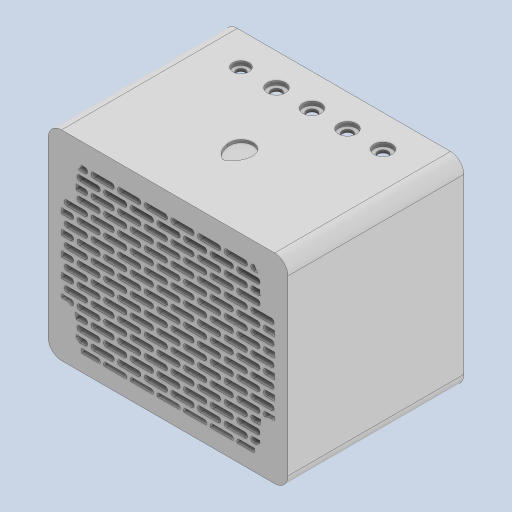
# Autodesk Inventor part: caixa_central
Saved by Autodesk Inventor 2023 (Build 270158000, 158)
## iProperties
Created: 2023-03-03
Part Number: caixa_central
Material: Genérico
Document SubType Name: Modeling
Designer: texugo
Density: 1 g/cm^3
Appearance: Padrão
Author: texugo
Autodesk Inventor part; units mm, degrees
(part 1 of 7)
ref_plane "YZ Plane" through (0, 0, 0) normal (1, 0, 0) x (0, 1, 0)
ref_plane "XZ Plane" through (0, 0, 0) normal (0, 1, 0) x (-1, 0, 0)
ref_plane "XY Plane" through (0, 0, 0) normal (0, 0, 1) x (1, 0, 0)
sketch "Esboço1" plane through (0, 0, 0) normal (0, 0, 1) x (1, 0, 0)
  line L0 (-75, 70) -> (75, 70)
  line L1 (85, 60) -> (85, -60)
  line L2 (75, -70) -> (-75, -70)
  line L3 (-85, -60) -> (-85, 60)
  line L4 (85, 70) -> (-85, -70) construction
  line L5 (-78, 73) -> (78, 73)
  line L6 (88, 63) -> (88, -63)
  line L7 (78, -73) -> (-78, -73)
  line L8 (-88, -63) -> (-88, 63)
  line L9 (-88, 73) -> (88, -73) construction
  arc A0 (-75, 70) -> (-85, 60) centre (-75, 60) ccw
  arc A1 (-78, 73) -> (-88, 63) centre (-78, 63) ccw
  arc A2 (85, 60) -> (75, 70) centre (75, 60) ccw
  arc A3 (88, 63) -> (78, 73) centre (78, 63) ccw
  arc A4 (75, -70) -> (85, -60) centre (75, -60) ccw
  arc A5 (78, -73) -> (88, -63) centre (78, -63) ccw
  arc A6 (-88, -63) -> (-78, -73) centre (-78, -63) ccw
  arc A7 (-85, -60) -> (-75, -70) centre (-75, -60) ccw
  circle A8 centre (-73.7339, -61.8573) radius 1.25
  line L10 (0, 0) -> (0, 1.4904)
  line L11 (0, 0) -> (1.3651, 0)
  line L12 (-73.7339, -52.8401) -> (-85, -52.8401)
  line L13 (-64.7396, -62.5) -> (-64.7396, -70)
  arc A9 (-64.7396, -62.5) -> (-74.5, -52.8727) centre (-73.7339, -61.8573) ccw
  circle A10 centre (73.7339, -61.8573) radius 1.25
  line L14 (73.7339, -52.8401) -> (85, -52.8401)
  line L15 (64.7396, -62.5) -> (64.7396, -70)
  arc A11 (74.5, -52.8727) -> (64.7396, -62.5) centre (73.7339, -61.8573) ccw
  line L16 (-80, -42) -> (-77, -42)
  circle A12 centre (-77, -42) radius 1.25
  arc A13 (-69.0044, -42.2652) -> (-77, -34) centre (-77, -42) ccw
  line L17 (-77, -34) -> (-85, -34)
  line L18 (-69, -42) -> (-69, -54.1827)
  circle A14 centre (77, -42) radius 1.25
  arc A15 (77, -34) -> (69.0044, -42.2652) centre (77, -42) ccw
  line L19 (69, -42) -> (69, -54.1827)
  arc A16 (-77, 34) -> (-69.0044, 42.2652) centre (-77, 42) ccw
  line L20 (-77, 34) -> (-85, 34)
  line L21 (-69, 42) -> (-69, 54.1827)
  arc A17 (69.0044, 42.2652) -> (77, 34) centre (77, 42) ccw
  line L22 (69, 42) -> (69, 54.1827)
  line L23 (77, -34) -> (85, -34)
  circle A18 centre (-73.7339, 61.8573) radius 1.25
  line L24 (-73.7339, 52.8401) -> (-85, 52.8401)
  line L25 (-64.7396, 62.5) -> (-64.7396, 70)
  arc A19 (-74.5, 52.8727) -> (-64.7396, 62.5) centre (-73.7339, 61.8573) ccw
  arc A20 (64.7396, 62.5) -> (74.5, 52.8727) centre (73.7339, 61.8573) ccw
  line L26 (64.7396, 62.5) -> (64.7396, 70)
  line L27 (73.7339, 52.8401) -> (85, 52.8401)
  circle A21 centre (73.7339, 61.8573) radius 1.25
  line L28 (77, 34) -> (85, 34)
  circle A22 centre (-73.7339, 61.8573) radius 1.25
  circle A23 centre (73.7339, 61.8573) radius 1.25
  circle A24 centre (-77, 42) radius 1.25
  circle A25 centre (77, 42) radius 1.25
  dimension "d4" = 10
  dimension "d8" = 2.5
  dimension "d12" = 3
  dimension "d13" = 2.5
  constraints: 58 end point, 44 symmetric about line, 41 point on circle, 26 centre point, 20 tangent, 11 point on line, 7 coincident, 7 equal radius, 5 perpendicular, 4 parallel, 3 horizontal, 2 midpoint, 2 vertical, 14 other
  measures "d4" radius of A0
  measures "d8" diameter of A8
  measures "d12" distance of L16.start L16.end
  measures "d13" diameter of A12
extrude "Extrusão1" add sketch "Esboço1" along normal blind 4 contours L0 L25 A19 L24 L3 A0 | L0 L26 A20 L22 A17 L28 L1 L23 A15 L19 A11 L15 L2 L13 A9 L18 A13 L17 L3 L20 A16 L21 A19 L25 | L0 A2 L1 L27 A20 L26 | L24 A19 L21 A16 L20 L3 | A20 L27 L1 L28 A17 L22 | L17 A13 L18 A9 L12 L3 | L12 A9 L13 L2 A7 L3 | L1 L14 A11 L19 A15 L23 | L1 A4 L2 L15 A11 L14 | L5 A3 L6 A5 L7 A6 L8 A1 | A8 | A10 | A12 | A14 | A18 | A21 | A24 | A25
sketch "Esboço2" plane through (0, 0, 0) normal (0, 0, -1) x (-1, 0, 0)
  line L0 (-75, 70) -> (75, 70)
  line L1 (85, 60) -> (85, -60)
  line L2 (75, -70) -> (-75, -70)
  line L3 (-85, -60) -> (-85, 60)
  line L4 (85, 70) -> (-85, -70) construction
  line L5 (-78, 73) -> (78, 73)
  line L6 (88, 63) -> (88, -63)
  line L7 (78, -73) -> (-78, -73)
  line L8 (-88, -63) -> (-88, 63)
  line L9 (-88, 73) -> (88, -73) construction
  arc A0 (-75, 70) -> (-85, 60) centre (-75, 60) ccw
  arc A1 (-78, 73) -> (-88, 63) centre (-78, 63) ccw
  arc A2 (85, 60) -> (75, 70) centre (75, 60) ccw
  arc A3 (88, 63) -> (78, 73) centre (78, 63) ccw
  arc A4 (75, -70) -> (85, -60) centre (75, -60) ccw
  arc A5 (78, -73) -> (88, -63) centre (78, -63) ccw
  arc A6 (-88, -63) -> (-78, -73) centre (-78, -63) ccw
  arc A7 (-85, -60) -> (-75, -70) centre (-75, -60) ccw
  circle A8 centre (-73.7339, -61.8573) radius 1.25
  line L10 (0, 0) -> (0, 1.4904)
  line L11 (0, 0) -> (1.3651, 0)
  line L12 (-73.7339, -52.8401) -> (-85, -52.8401)
  line L13 (-64.7396, -62.5) -> (-64.7396, -70)
  arc A9 (-64.7396, -62.5) -> (-74.5, -52.8727) centre (-73.7339, -61.8573) ccw
  arc A10 (74.5, -52.8727) -> (64.7396, -62.5) centre (73.7339, -61.8573) ccw
  line L14 (64.7396, -62.5) -> (64.7396, -70)
  line L15 (73.7339, -52.8401) -> (85, -52.8401)
  circle A11 centre (73.7339, -61.8573) radius 1.25
  line L16 (-80, -42) -> (-77, -42)
  circle A12 centre (-77, -42) radius 1.25
  arc A13 (-69.0044, -42.2652) -> (-77, -34) centre (-77, -42) ccw
  line L17 (-77, -34) -> (-85, -34)
  line L18 (-69, -42) -> (-69, -54.1827)
  arc A14 (77, -34) -> (69.0044, -42.2652) centre (77, -42) ccw
  line L19 (69, -42) -> (69, -54.1827)
  circle A15 centre (77, -42) radius 1.25
  line L20 (-77, 34) -> (-85, 34)
  arc A16 (-77, 34) -> (-69.0044, 42.2652) centre (-77, 42) ccw
  line L21 (-69, 42) -> (-69, 54.1827)
  line L22 (69, 42) -> (69, 54.1827)
  arc A17 (69.0044, 42.2652) -> (77, 34) centre (77, 42) ccw
  line L23 (77, -34) -> (85, -34)
  line L24 (77, 34) -> (85, 34)
  line L25 (64.7396, 62.5) -> (64.7396, 70)
  arc A18 (64.7396, 62.5) -> (74.5, 52.8727) centre (73.7339, 61.8573) ccw
  line L26 (73.7339, 52.8401) -> (85, 52.8401)
  circle A19 centre (73.7339, 61.8573) radius 1.25
  line L27 (-64.7396, 62.5) -> (-64.7396, 70)
  arc A20 (-74.5, 52.8727) -> (-64.7396, 62.5) centre (-73.7339, 61.8573) ccw
  circle A21 centre (-73.7339, 61.8573) radius 1.25
  line L28 (-73.7339, 52.8401) -> (-85, 52.8401)
  circle A22 centre (-73.7339, 61.8573) radius 1.25
  circle A23 centre (73.7339, 61.8573) radius 1.25
  circle A24 centre (77, 42) radius 1.25
  circle A25 centre (-77, 42) radius 1.25
  dimension "d16" = 10
  dimension "d17" = 2.5
  dimension "d18" = 3
  dimension "d19" = 2.5
  constraints: 58 end point, 44 symmetric about line, 41 point on circle, 26 centre point, 20 tangent, 11 point on line, 7 coincident, 7 equal radius, 5 perpendicular, 4 parallel, 3 horizontal, 2 midpoint, 2 vertical, 14 other
  measures "d16" radius of A0
  measures "d17" diameter of A8
  measures "d18" distance of L16.start L16.end
  measures "d19" diameter of A12
extrude "Extrusão2" add sketch "Esboço2" along normal blind 10 contours L0 L27 A20 L28 L3 A0 | L0 A2 L1 L26 A18 L25 | L28 A20 L21 A16 L20 L3 | A18 L26 L1 L24 A17 L22 | L17 A13 L18 A9 L12 L3 | L12 A9 L13 L2 A7 L3 | L1 L15 A10 L19 A14 L23 | L1 A4 L2 L14 A10 L15 | L5 A3 L6 A5 L7 A6 L8 A1 | A8 | A11 | A12 | A15 | A19 | A21 | A24 | A25
sketch "Esboço3" plane through (0, 0, -10) normal (0, 0, -1) x (-1, 0, 0)
  line L0 (-75, 70) -> (75, 70)
  line L1 (85, 60) -> (85, -60)
  line L2 (75, -70) -> (-75, -70)
  line L3 (-85, -60) -> (-85, 60)
  line L4 (85, 70) -> (-85, -70) construction
  line L5 (-78, 73) -> (78, 73)
  line L6 (88, 63) -> (88, -63)
  line L7 (78, -73) -> (-78, -73)
  line L8 (-88, -63) -> (-88, 63)
  line L9 (-88, 73) -> (88, -73) construction
  arc A0 (-75, 70) -> (-85, 60) centre (-75, 60) ccw
  arc A1 (-78, 73) -> (-88, 63) centre (-78, 63) ccw
  arc A2 (85, 60) -> (75, 70) centre (75, 60) ccw
  arc A3 (88, 63) -> (78, 73) centre (78, 63) ccw
  arc A4 (75, -70) -> (85, -60) centre (75, -60) ccw
  arc A5 (78, -73) -> (88, -63) centre (78, -63) ccw
  arc A6 (-88, -63) -> (-78, -73) centre (-78, -63) ccw
  arc A7 (-85, -60) -> (-75, -70) centre (-75, -60) ccw
  circle A8 centre (-73.7339, -61.8573) radius 1.25
  line L10 (0, 0) -> (0, 1.4904)
  line L11 (0, 0) -> (1.3651, 0)
  line L12 (-73.7339, -52.8401) -> (-85, -52.8401)
  line L13 (-64.7396, -62.5) -> (-64.7396, -70)
  arc A9 (-64.7396, -62.5) -> (-74.5, -52.8727) centre (-73.7339, -61.8573) ccw
  arc A10 (74.5, -52.8727) -> (64.7396, -62.5) centre (73.7339, -61.8573) ccw
  line L14 (64.7396, -62.5) -> (64.7396, -70)
  line L15 (73.7339, -52.8401) -> (85, -52.8401)
  circle A11 centre (73.7339, -61.8573) radius 1.25
  line L16 (-80, -42) -> (-77, -42)
  circle A12 centre (-77, -42) radius 1.25
  arc A13 (-69.0044, -42.2652) -> (-77, -34) centre (-77, -42) ccw
  line L17 (-77, -34) -> (-85, -34)
  line L18 (-69, -42) -> (-69, -54.1827)
  arc A14 (77, -34) -> (69.0044, -42.2652) centre (77, -42) ccw
  line L19 (69, -42) -> (69, -54.1827)
  circle A15 centre (77, -42) radius 1.25
  line L20 (-77, 34) -> (-85, 34)
  arc A16 (-77, 34) -> (-69.0044, 42.2652) centre (-77, 42) ccw
  line L21 (-69, 42) -> (-69, 54.1827)
  line L22 (69, 42) -> (69, 54.1827)
  arc A17 (69.0044, 42.2652) -> (77, 34) centre (77, 42) ccw
  line L23 (77, -34) -> (85, -34)
  line L24 (77, 34) -> (85, 34)
  line L25 (64.7396, 62.5) -> (64.7396, 70)
  arc A18 (64.7396, 62.5) -> (74.5, 52.8727) centre (73.7339, 61.8573) ccw
  line L26 (73.7339, 52.8401) -> (85, 52.8401)
  circle A19 centre (73.7339, 61.8573) radius 1.25
  line L27 (-64.7396, 62.5) -> (-64.7396, 70)
  arc A20 (-74.5, 52.8727) -> (-64.7396, 62.5) centre (-73.7339, 61.8573) ccw
  circle A21 centre (-73.7339, 61.8573) radius 1.25
  line L28 (-73.7339, 52.8401) -> (-85, 52.8401)
  circle A22 centre (-73.7339, 61.8573) radius 1.25
  circle A23 centre (73.7339, 61.8573) radius 1.25
  circle A24 centre (77, 42) radius 1.25
  circle A25 centre (-77, 42) radius 1.25
  dimension "d22" = 10
  dimension "d23" = 2.5
  dimension "d24" = 3
  dimension "d25" = 2.5
  constraints: 58 end point, 44 symmetric about line, 41 point on circle, 26 centre point, 20 tangent, 11 point on line, 7 coincident, 7 equal radius, 5 perpendicular, 4 parallel, 3 horizontal, 2 midpoint, 2 vertical, 14 other
  measures "d22" radius of A0
  measures "d23" diameter of A8
  measures "d24" distance of L16.start L16.end
  measures "d25" diameter of A12
extrude "Extrusão3" cut sketch "Esboço3" against normal blind 5 contours A12 | A15 | A24 | A25
sketch "Esboço4" plane through (0, 0, -10) normal (0, 0, -1) x (-1, 0, 0)
  line L0 (-75, 70) -> (75, 70)
  line L1 (85, 60) -> (85, -60)
  line L2 (75, -70) -> (-75, -70)
  line L3 (-85, -60) -> (-85, 60)
  line L4 (85, 70) -> (-85, -70) construction
  line L5 (-78, 73) -> (78, 73)
  line L6 (88, 63) -> (88, -63)
  line L7 (78, -73) -> (-78, -73)
  line L8 (-88, -63) -> (-88, 63)
  line L9 (-88, 73) -> (88, -73) construction
  arc A0 (-75, 70) -> (-85, 60) centre (-75, 60) ccw
  arc A1 (-78, 73) -> (-88, 63) centre (-78, 63) ccw
  arc A2 (85, 60) -> (75, 70) centre (75, 60) ccw
  arc A3 (88, 63) -> (78, 73) centre (78, 63) ccw
  arc A4 (75, -70) -> (85, -60) centre (75, -60) ccw
  arc A5 (78, -73) -> (88, -63) centre (78, -63) ccw
  arc A6 (-88, -63) -> (-78, -73) centre (-78, -63) ccw
  arc A7 (-85, -60) -> (-75, -70) centre (-75, -60) ccw
  circle A8 centre (-73.7339, -61.8573) radius 1.25
  line L10 (0, 0) -> (0, 1.4904)
  line L11 (0, 0) -> (1.3651, 0)
  line L12 (-73.7339, -52.8401) -> (-85, -52.8401)
  line L13 (-64.7396, -62.5) -> (-64.7396, -70)
  arc A9 (-64.7396, -62.5) -> (-74.5, -52.8727) centre (-73.7339, -61.8573) ccw
  arc A10 (74.5, -52.8727) -> (64.7396, -62.5) centre (73.7339, -61.8573) ccw
  line L14 (64.7396, -62.5) -> (64.7396, -70)
  line L15 (73.7339, -52.8401) -> (85, -52.8401)
  circle A11 centre (73.7339, -61.8573) radius 1.25
  line L16 (-80, -42) -> (-77, -42)
  circle A12 centre (-77, -42) radius 1.25
  arc A13 (-69.0044, -42.2652) -> (-77, -34) centre (-77, -42) ccw
  line L17 (-77, -34) -> (-85, -34)
  line L18 (-69, -42) -> (-69, -54.1827)
  arc A14 (77, -34) -> (69.0044, -42.2652) centre (77, -42) ccw
  line L19 (69, -42) -> (69, -54.1827)
  circle A15 centre (77, -42) radius 1.25
  line L20 (-77, 34) -> (-85, 34)
  arc A16 (-77, 34) -> (-69.0044, 42.2652) centre (-77, 42) ccw
  line L21 (-69, 42) -> (-69, 54.1827)
  line L22 (69, 42) -> (69, 54.1827)
  arc A17 (69.0044, 42.2652) -> (77, 34) centre (77, 42) ccw
  line L23 (77, -34) -> (85, -34)
  line L24 (77, 34) -> (85, 34)
  line L25 (64.7396, 62.5) -> (64.7396, 70)
  arc A18 (64.7396, 62.5) -> (74.5, 52.8727) centre (73.7339, 61.8573) ccw
  line L26 (73.7339, 52.8401) -> (85, 52.8401)
  circle A19 centre (73.7339, 61.8573) radius 1.25
  line L27 (-64.7396, 62.5) -> (-64.7396, 70)
  arc A20 (-74.5, 52.8727) -> (-64.7396, 62.5) centre (-73.7339, 61.8573) ccw
  circle A21 centre (-73.7339, 61.8573) radius 1.25
  line L28 (-73.7339, 52.8401) -> (-85, 52.8401)
  circle A22 centre (-73.7339, 61.8573) radius 1.25
  circle A23 centre (73.7339, 61.8573) radius 1.25
  circle A24 centre (77, 42) radius 1.25
  circle A25 centre (-77, 42) radius 1.25
  dimension "d28" = 10
  dimension "d29" = 2.5
  dimension "d30" = 3
  dimension "d31" = 2.5
  constraints: 58 end point, 44 symmetric about line, 41 point on circle, 26 centre point, 20 tangent, 11 point on line, 7 coincident, 7 equal radius, 5 perpendicular, 4 parallel, 3 horizontal, 2 midpoint, 2 vertical, 14 other
  measures "d28" radius of A0
  measures "d29" diameter of A8
  measures "d30" distance of L16.start L16.end
  measures "d31" diameter of A12
extrude "Extrusão4" add sketch "Esboço4" along normal blind 70 contours L0 L27 A20 L28 L3 A0 | L0 A2 L1 L26 A18 L25 | L12 A9 L13 L2 A7 L3 | L1 A4 L2 L14 A10 L15 | L5 A3 L6 A5 L7 A6 L8 A1 | A8 | A11 | A19 | A21
sketch "Esboço5" plane through (0, 0, -80) normal (0, 0, -1) x (-1, 0, 0)
  line L0 (-75, 70) -> (75, 70)
  line L1 (85, 60) -> (85, -60)
  line L2 (75, -70) -> (-75, -70)
  line L3 (-85, -60) -> (-85, 60)
  line L4 (85, 70) -> (-85, -70) construction
  line L5 (-78, 73) -> (78, 73)
  line L6 (88, 63) -> (88, -63)
  line L7 (78, -73) -> (-78, -73)
  line L8 (-88, -63) -> (-88, 63)
  line L9 (-88, 73) -> (88, -73) construction
  arc A0 (-75, 70) -> (-85, 60) centre (-75, 60) ccw
  arc A1 (-78, 73) -> (-88, 63) centre (-78, 63) ccw
  arc A2 (85, 60) -> (75, 70) centre (75, 60) ccw
  arc A3 (88, 63) -> (78, 73) centre (78, 63) ccw
  arc A4 (75, -70) -> (85, -60) centre (75, -60) ccw
  arc A5 (78, -73) -> (88, -63) centre (78, -63) ccw
  arc A6 (-88, -63) -> (-78, -73) centre (-78, -63) ccw
  arc A7 (-85, -60) -> (-75, -70) centre (-75, -60) ccw
  circle A8 centre (-73.7339, -61.8573) radius 1.25
  line L10 (0, 0) -> (0, 1.4904)
  line L11 (0, 0) -> (1.3651, 0)
  line L12 (-73.7339, -52.8401) -> (-85, -52.8401)
  line L13 (-64.7396, -62.5) -> (-64.7396, -70)
  arc A9 (-64.7396, -62.5) -> (-74.5, -52.8727) centre (-73.7339, -61.8573) ccw
  arc A10 (74.5, -52.8727) -> (64.7396, -62.5) centre (73.7339, -61.8573) ccw
  line L14 (64.7396, -62.5) -> (64.7396, -70)
  line L15 (73.7339, -52.8401) -> (85, -52.8401)
  circle A11 centre (73.7339, -61.8573) radius 1.25
  line L16 (-80, -42) -> (-77, -42)
  circle A12 centre (-77, -42) radius 1.25
  arc A13 (-69.0044, -42.2652) -> (-77, -34) centre (-77, -42) ccw
  line L17 (-77, -34) -> (-85, -34)
  line L18 (-69, -42) -> (-69, -54.1827)
  arc A14 (77, -34) -> (69.0044, -42.2652) centre (77, -42) ccw
  line L19 (69, -42) -> (69, -54.1827)
  circle A15 centre (77, -42) radius 1.25
  line L20 (-77, 34) -> (-85, 34)
  arc A16 (-77, 34) -> (-69.0044, 42.2652) centre (-77, 42) ccw
  line L21 (-69, 42) -> (-69, 54.1827)
  line L22 (69, 42) -> (69, 54.1827)
  arc A17 (69.0044, 42.2652) -> (77, 34) centre (77, 42) ccw
  line L23 (77, -34) -> (85, -34)
  line L24 (77, 34) -> (85, 34)
  line L25 (64.7396, 62.5) -> (64.7396, 70)
  arc A18 (64.7396, 62.5) -> (74.5, 52.8727) centre (73.7339, 61.8573) ccw
  line L26 (73.7339, 52.8401) -> (85, 52.8401)
  circle A19 centre (73.7339, 61.8573) radius 1.25
  line L27 (-64.7396, 62.5) -> (-64.7396, 70)
  arc A20 (-74.5, 52.8727) -> (-64.7396, 62.5) centre (-73.7339, 61.8573) ccw
  circle A21 centre (-73.7339, 61.8573) radius 1.25
  line L28 (-73.7339, 52.8401) -> (-85, 52.8401)
  circle A22 centre (-73.7339, 61.8573) radius 1.25
  circle A23 centre (73.7339, 61.8573) radius 1.25
  circle A24 centre (77, 42) radius 1.25
  circle A25 centre (-77, 42) radius 1.25
  dimension "d34" = 10
  dimension "d35" = 2.5
  dimension "d36" = 3
  dimension "d37" = 2.5
  constraints: 58 end point, 44 symmetric about line, 41 point on circle, 26 centre point, 20 tangent, 11 point on line, 7 coincident, 7 equal radius, 5 perpendicular, 4 parallel, 3 horizontal, 2 midpoint, 2 vertical, 14 other
  measures "d34" radius of A0
  measures "d35" diameter of A8
  measures "d36" distance of L16.start L16.end
  measures "d37" diameter of A12
extrude "Extrusão5" cut sketch "Esboço5" against normal blind 7 contours A8 | A11 | A19 | A21
sketch "Esboço6" plane through (0, 0, -80) normal (0, 0, -1) x (-1, 0, 0)
  line L0 (-75, 70) -> (75, 70)
  line L1 (85, 60) -> (85, -60)
  line L2 (75, -70) -> (-75, -70)
  line L3 (-85, -60) -> (-85, 60)
  line L4 (85, 70) -> (-85, -70) construction
  line L5 (-78, 73) -> (78, 73)
  line L6 (88, 63) -> (88, -63)
  line L7 (78, -73) -> (-78, -73)
  line L8 (-88, -63) -> (-88, 63)
  line L9 (-88, 73) -> (88, -73) construction
  arc A0 (-75, 70) -> (-85, 60) centre (-75, 60) ccw
  arc A1 (-78, 73) -> (-88, 63) centre (-78, 63) ccw
  arc A2 (85, 60) -> (75, 70) centre (75, 60) ccw
  arc A3 (88, 63) -> (78, 73) centre (78, 63) ccw
  arc A4 (75, -70) -> (85, -60) centre (75, -60) ccw
  arc A5 (78, -73) -> (88, -63) centre (78, -63) ccw
  arc A6 (-88, -63) -> (-78, -73) centre (-78, -63) ccw
  arc A7 (-85, -60) -> (-75, -70) centre (-75, -60) ccw
  circle A8 centre (-73.7339, -61.8573) radius 1.25
  line L10 (0, 0) -> (0, 1.4904)
  line L11 (0, 0) -> (1.3651, 0)
  line L12 (-73.7339, -52.8401) -> (-85, -52.8401)
  line L13 (-64.7396, -62.5) -> (-64.7396, -70)
  arc A9 (-64.7396, -62.5) -> (-74.5, -52.8727) centre (-73.7339, -61.8573) ccw
  arc A10 (74.5, -52.8727) -> (64.7396, -62.5) centre (73.7339, -61.8573) ccw
  line L14 (64.7396, -62.5) -> (64.7396, -70)
  line L15 (73.7339, -52.8401) -> (85, -52.8401)
  circle A11 centre (73.7339, -61.8573) radius 1.25
  line L16 (-80, -42) -> (-77, -42)
  circle A12 centre (-77, -42) radius 1.25
  arc A13 (-69.0044, -42.2652) -> (-77, -34) centre (-77, -42) ccw
  line L17 (-77, -34) -> (-85, -34)
  line L18 (-69, -42) -> (-69, -54.1827)
  arc A14 (77, -34) -> (69.0044, -42.2652) centre (77, -42) ccw
  line L19 (69, -42) -> (69, -54.1827)
  circle A15 centre (77, -42) radius 1.25
  line L20 (-77, 34) -> (-85, 34)
  arc A16 (-77, 34) -> (-69.0044, 42.2652) centre (-77, 42) ccw
  line L21 (-69, 42) -> (-69, 54.1827)
  line L22 (69, 42) -> (69, 54.1827)
  arc A17 (69.0044, 42.2652) -> (77, 34) centre (77, 42) ccw
  line L23 (77, -34) -> (85, -34)
  line L24 (77, 34) -> (85, 34)
  line L25 (64.7396, 62.5) -> (64.7396, 70)
  arc A18 (64.7396, 62.5) -> (74.5, 52.8727) centre (73.7339, 61.8573) ccw
  line L26 (73.7339, 52.8401) -> (85, 52.8401)
  circle A19 centre (73.7339, 61.8573) radius 1.25
  line L27 (-64.7396, 62.5) -> (-64.7396, 70)
  arc A20 (-74.5, 52.8727) -> (-64.7396, 62.5) centre (-73.7339, 61.8573) ccw
  circle A21 centre (-73.7339, 61.8573) radius 1.25
  line L28 (-73.7339, 52.8401) -> (-85, 52.8401)
  circle A22 centre (-73.7339, 61.8573) radius 1.25
  circle A23 centre (73.7339, 61.8573) radius 1.25
  circle A24 centre (77, 42) radius 1.25
  circle A25 centre (-77, 42) radius 1.25
  dimension "d40" = 10
  dimension "d41" = 2.5
  dimension "d42" = 3
  dimension "d43" = 2.5
  constraints: 58 end point, 44 symmetric about line, 41 point on circle, 26 centre point, 20 tangent, 11 point on line, 7 coincident, 7 equal radius, 5 perpendicular, 4 parallel, 3 horizontal, 2 midpoint, 2 vertical, 14 other
  measures "d40" radius of A0
  measures "d41" diameter of A8
  measures "d42" distance of L16.start L16.end
  measures "d43" diameter of A12
extrude "Extrusão6" add sketch "Esboço6" along normal blind 45 contours L5 A3 L6 A5 L7 A6 L8 A1
sketch "Esboço7" plane through (0, 0, 0) normal (0, 0, 1) x (1, 0, 0)
  line L0 (80, 75) -> (-80, 75)
  line L1 (-90, 65) -> (-90, -65)
  line L2 (-80, -75) -> (80, -75)
  line L3 (90, -65) -> (90, 65)
  line L4 (90, 75) -> (-90, -75) construction
  line L5 (-90, 75) -> (90, -75) construction
  arc A0 (80, -75) -> (90, -65) centre (80, -65) ccw
  arc A1 (-90, -65) -> (-80, -75) centre (-80, -65) ccw
  arc A2 (-80, 75) -> (-90, 65) centre (-80, 65) ccw
  arc A3 (90, 65) -> (80, 75) centre (80, 65) ccw
  line L6 (-75, 70) -> (75, 70)
  line L7 (85, 60) -> (85, -60)
  line L8 (75, -70) -> (-75, -70)
  line L9 (-85, -60) -> (-85, 60)
  line L10 (85, 70) -> (-85, -70) construction
  line L11 (-78, 73) -> (78, 73)
  line L12 (88, 63) -> (88, -63)
  line L13 (78, -73) -> (-78, -73)
  line L14 (-88, -63) -> (-88, 63)
  line L15 (-88, 73) -> (88, -73) construction
  arc A4 (-75, 70) -> (-85, 60) centre (-75, 60) ccw
  arc A5 (-78, 73) -> (-88, 63) centre (-78, 63) ccw
  arc A6 (85, 60) -> (75, 70) centre (75, 60) ccw
  arc A7 (88, 63) -> (78, 73) centre (78, 63) ccw
  arc A8 (75, -70) -> (85, -60) centre (75, -60) ccw
  arc A9 (78, -73) -> (88, -63) centre (78, -63) ccw
  arc A10 (-88, -63) -> (-78, -73) centre (-78, -63) ccw
  arc A11 (-85, -60) -> (-75, -70) centre (-75, -60) ccw
  circle A12 centre (-73.7339, -61.8573) radius 1.25
  line L16 (0, 0) -> (0, 1.4904)
  line L17 (0, 0) -> (1.3651, 0)
  line L18 (-73.7339, -52.8401) -> (-85, -52.8401)
  line L19 (-64.7396, -62.5) -> (-64.7396, -70)
  arc A13 (-64.7396, -62.5) -> (-74.5, -52.8727) centre (-73.7339, -61.8573) ccw
  arc A14 (74.5, -52.8727) -> (64.7396, -62.5) centre (73.7339, -61.8573) ccw
  line L20 (64.7396, -62.5) -> (64.7396, -70)
  line L21 (73.7339, -52.8401) -> (85, -52.8401)
  circle A15 centre (73.7339, -61.8573) radius 1.25
  line L22 (-80, -42) -> (-77, -42)
  circle A16 centre (-77, -42) radius 1.25
  arc A17 (-69.0044, -42.2652) -> (-77, -34) centre (-77, -42) ccw
  line L23 (-77, -34) -> (-85, -34)
  line L24 (-69, -42) -> (-69, -54.1827)
  arc A18 (77, -34) -> (69.0044, -42.2652) centre (77, -42) ccw
  line L25 (69, -42) -> (69, -54.1827)
  circle A19 centre (77, -42) radius 1.25
  line L26 (-77, 34) -> (-85, 34)
  arc A20 (-77, 34) -> (-69.0044, 42.2652) centre (-77, 42) ccw
  line L27 (-69, 42) -> (-69, 54.1827)
  line L28 (69, 42) -> (69, 54.1827)
  arc A21 (69.0044, 42.2652) -> (77, 34) centre (77, 42) ccw
  line L29 (77, -34) -> (85, -34)
  line L30 (77, 34) -> (85, 34)
  line L31 (64.7396, 62.5) -> (64.7396, 70)
  arc A22 (64.7396, 62.5) -> (74.5, 52.8727) centre (73.7339, 61.8573) ccw
  line L32 (73.7339, 52.8401) -> (85, 52.8401)
  circle A23 centre (73.7339, 61.8573) radius 1.25
  line L33 (-64.7396, 62.5) -> (-64.7396, 70)
  arc A24 (-74.5, 52.8727) -> (-64.7396, 62.5) centre (-73.7339, 61.8573) ccw
  circle A25 centre (-73.7339, 61.8573) radius 1.25
  line L34 (-73.7339, 52.8401) -> (-85, 52.8401)
  circle A26 centre (-73.7339, 61.8573) radius 1.25
  circle A27 centre (73.7339, 61.8573) radius 1.25
  circle A28 centre (77, 42) radius 1.25
  circle A29 centre (-77, 42) radius 1.25
  dimension "d46" = 180
  dimension "d47" = 150
  dimension "d48" = 10
  dimension "d49" = 10
  dimension "d50" = 2.5
  dimension "d51" = 3
  dimension "d52" = 2.5
  constraints: 70 end point, 49 point on circle, 44 symmetric about line, 30 centre point, 28 tangent, 19 point on line, 10 equal radius, 7 coincident, 6 parallel, 6 perpendicular, 4 horizontal, 4 midpoint, 2 vertical, 14 other
  measures "d46" distance of L5.end L4.end
  measures "d47" distance of L4.end L5.start
  measures "d48" radius of A0
  measures "d49" radius of A4
  measures "d50" diameter of A12
  measures "d51" distance of L22.start L22.end
  measures "d52" diameter of A16
extrude "Extrusão7" add sketch "Esboço7" along normal blind 4 and the other way blind 128 contours A3 L3 A0 L2 A1 L1 A2 L0
sketch "Esboço8" plane through (0, 0, -125) normal (0, 0, -1) x (-1, 0, 0)
  arc A0 (-78, 73) -> (-88, 63) centre (-78, 63) ccw
  arc A1 (-78, 73) -> (-88, 63) centre (-78, 63) ccw
  line L0 (-85.0711, 70.0711) -> (-80.8284, 65.8284)
  line L1 (-85.0711, 70.0711) -> (-79.0711, 70.0711) construction
  circle A2 centre (-80.8284, 65.8284) radius 1
  line L2 (-88, 63) -> (-88, -63)
  line L3 (0, 0) -> (0, 9)
  line L4 (0, 0) -> (10, 0)
  circle A3 centre (80.8284, 65.8284) radius 1
  line L5 (85.0711, 70.0711) -> (79.0711, 70.0711) construction
  arc A4 (88, 63) -> (78, 73) centre (78, 63) ccw
  arc A5 (88, 63) -> (78, 73) centre (78, 63) ccw
  circle A6 centre (-80.8284, -65.8284) radius 1
  line L6 (-85.0711, -70.0711) -> (-79.0711, -70.0711) construction
  arc A7 (-88, -63) -> (-78, -73) centre (-78, -63) ccw
  arc A8 (-88, -63) -> (-78, -73) centre (-78, -63) ccw
  circle A9 centre (80.8284, -65.8284) radius 1
  line L7 (85.0711, -70.0711) -> (79.0711, -70.0711) construction
  arc A10 (78, -73) -> (88, -63) centre (78, -63) ccw
  arc A11 (78, -73) -> (88, -63) centre (78, -63) ccw
  line L8 (-80, 49) -> (80, 49)
  line L9 (80, 49) -> (80, -49)
  line L10 (80, -49) -> (-80, -49)
  line L11 (-80, -49) -> (-80, 49)
  line L12 (-80, 49) -> (80, -49) construction
  line L13 (80, 49) -> (-80, -49) construction
  line L14 (-75, 62.5) -> (75, 62.5)
  line L15 (75, 62.5) -> (75, -62.5)
  line L16 (75, -62.5) -> (-75, -62.5)
  line L17 (-75, -62.5) -> (-75, 62.5)
  line L18 (-75, 62.5) -> (75, -62.5) construction
  line L19 (75, 62.5) -> (-75, -62.5) construction
  line L20 (-88, -63) -> (-88, 63)
  arc A12 (-78, 73) -> (-88, 63) centre (-78, 63) ccw
  arc A13 (-88, 63) -> (-78, 73) centre (-82.7974, 67.7974) ccw
  arc A14 (78, 73) -> (88, 63) centre (82.7974, 67.7974) ccw
  arc A15 (-78, -73) -> (-88, -63) centre (-82.7974, -67.7974) ccw
  arc A16 (88, -63) -> (78, -73) centre (82.7974, -67.7974) ccw
  dimension "d77" = 6
  dimension "d78" = 45
  dimension "d79" = 2
  dimension "d80" = 160
  dimension "d81" = 98
  dimension "d82" = 150
  dimension "d83" = 125
  constraints: 42 end point, 27 point on circle, 26 symmetric about line, 17 centre point, 4 coincident, 4 horizontal, 4 midpoint, 4 parallel, 2 perpendicular, 1 equal length, 1 vertical, 12 other
  measures "d77" distance of L0.start L0.end
  measures "d78" angle of L0 L1
  measures "d79" diameter of A2
  measures "d80" distance of L9.end L10.end
  measures "d81" distance of L8.end L9.end
  measures "d82" distance of L15.end L16.end
  measures "d83" distance of L14.end L15.end
extrude "Extrusão8" add sketch "Esboço8" against normal blind 128 contours A13 A0 | A2 | A3 | A14 A4 | A6 | A15 A7 | A9 | A16 A10
sketch "Esboço9" plane through (0, 0, -125) normal (0, 0, -1) x (-1, 0, 0)
  arc A0 (-78, 73) -> (-88, 63) centre (-78, 63) ccw
  arc A1 (-78, 73) -> (-88, 63) centre (-78, 63) ccw
  line L0 (-85.0711, 70.0711) -> (-80.8284, 65.8284)
  line L1 (-85.0711, 70.0711) -> (-79.0711, 70.0711) construction
  circle A2 centre (-80.8284, 65.8284) radius 1
  line L2 (-88, 63) -> (-88, -63)
  line L3 (0, 0) -> (0, 9)
  line L4 (0, 0) -> (10, 0)
  circle A3 centre (80.8284, 65.8284) radius 1
  line L5 (85.0711, 70.0711) -> (79.0711, 70.0711) construction
  arc A4 (88, 63) -> (78, 73) centre (78, 63) ccw
  arc A5 (88, 63) -> (78, 73) centre (78, 63) ccw
  circle A6 centre (-80.8284, -65.8284) radius 1
  line L6 (-85.0711, -70.0711) -> (-79.0711, -70.0711) construction
  arc A7 (-88, -63) -> (-78, -73) centre (-78, -63) ccw
  arc A8 (-88, -63) -> (-78, -73) centre (-78, -63) ccw
  circle A9 centre (80.8284, -65.8284) radius 1
  line L7 (85.0711, -70.0711) -> (79.0711, -70.0711) construction
  arc A10 (78, -73) -> (88, -63) centre (78, -63) ccw
  arc A11 (78, -73) -> (88, -63) centre (78, -63) ccw
  line L8 (-80, 49) -> (80, 49)
  line L9 (80, 49) -> (80, -49)
  line L10 (80, -49) -> (-80, -49)
  line L11 (-80, -49) -> (-80, 49)
  line L12 (-80, 49) -> (80, -49) construction
  line L13 (80, 49) -> (-80, -49) construction
  line L14 (-75, 62.5) -> (75, 62.5)
  line L15 (75, 62.5) -> (75, -62.5)
  line L16 (75, -62.5) -> (-75, -62.5)
  line L17 (-75, -62.5) -> (-75, 62.5)
  line L18 (-75, 62.5) -> (75, -62.5) construction
  line L19 (75, 62.5) -> (-75, -62.5) construction
  line L20 (-88, -63) -> (-88, 63) projected
  arc A12 (-78, 73) -> (-88, 63) centre (-78, 63) ccw projected
  arc A13 (-88, 63) -> (-78, 73) centre (-82.7974, 67.7974) ccw
  arc A14 (78, 73) -> (88, 63) centre (82.7974, 67.7974) ccw
  arc A15 (-78, -73) -> (-88, -63) centre (-82.7974, -67.7974) ccw
  arc A16 (88, -63) -> (78, -73) centre (82.7974, -67.7974) ccw
  dimension "d66" = 6
  dimension "d67" = 45
  dimension "d68" = 2
  dimension "d73" = 160
  dimension "d74" = 98
  dimension "d75" = 150
  dimension "d76" = 125
  constraints: 40 end point, 26 symmetric about line, 25 point on circle, 16 centre point, 4 coincident, 4 horizontal, 4 midpoint, 4 parallel, 2 perpendicular, 1 equal length, 1 vertical, 12 other
  measures "d66" distance of L0.start L0.end
  measures "d67" angle of L0 L1
  measures "d68" diameter of A2
  measures "d73" distance of L9.end L10.end
  measures "d74" distance of L8.end L9.end
  measures "d75" distance of L15.end L16.end
  measures "d76" distance of L14.end L15.end
extrude "Extrusão9" cut sketch "Esboço9" against normal blind 6 contours A2 | A3 | A6 | A9
sketch "Esboço10" plane through (0, 0, 4) normal (0, 0, 1) x (1, 0, 0)
  line L0 (70, -62.5) -> (-70, -62.5)
  line L1 (-80, -52.5) -> (-80, 52.5)
  line L2 (-70, 62.5) -> (70, 62.5)
  line L3 (80, 52.5) -> (80, -52.5)
  arc A0 (70, -62.5) -> (80, -52.5) centre (70, -52.5) ccw
  arc A1 (80, 52.5) -> (70, 62.5) centre (70, 52.5) ccw
  arc A2 (-70, 62.5) -> (-80, 52.5) centre (-70, 52.5) ccw
  arc A3 (-80, -52.5) -> (-70, -62.5) centre (-70, -52.5) ccw
  line L4 (47.0881, -59.4916) -> (33.6537, -59.4916)
  line L5 (33.6537, -63.4916) -> (47.0881, -63.4916)
  arc A4 (47.0881, -63.4916) -> (47.0881, -59.4916) centre (47.0881, -61.4916) ccw
  arc A5 (33.6537, -59.4916) -> (33.6537, -63.4916) centre (33.6537, -61.4916) ccw
  line L6 (27.0881, -59.4916) -> (13.6537, -59.4916)
  line L7 (13.6537, -63.4916) -> (27.0881, -63.4916)
  arc A6 (27.0881, -63.4916) -> (27.0881, -59.4916) centre (27.0881, -61.4916) ccw
  arc A7 (13.6537, -59.4916) -> (13.6537, -63.4916) centre (13.6537, -61.4916) ccw
  arc A8 (44.1532, -52.5346) -> (44.1532, -56.5346) centre (44.1532, -54.5346) ccw
  line L8 (44.1532, -56.5346) -> (57.5876, -56.5346)
  arc A9 (57.5876, -56.5346) -> (57.5876, -52.5346) centre (57.5876, -54.5346) ccw
  arc A10 (24.1532, -52.5346) -> (24.1532, -56.5346) centre (24.1532, -54.5346) ccw
  line L9 (24.1532, -56.5346) -> (37.5876, -56.5346)
  line L10 (37.5876, -52.5346) -> (24.1532, -52.5346)
  arc A11 (37.5876, -56.5346) -> (37.5876, -52.5346) centre (37.5876, -54.5346) ccw
  arc A12 (44.1532, -52.5346) -> (44.1532, -56.5346) centre (44.1532, -54.5346) ccw
  line L11 (57.5876, -52.5346) -> (44.1532, -52.5346)
  arc A13 (-6.3463, -59.4916) -> (-6.3463, -63.4916) centre (-6.3463, -61.4916) ccw
  arc A14 (27.0881, -63.4916) -> (27.0881, -59.4916) centre (27.0881, -61.4916) ccw
  arc A15 (24.1532, -52.5346) -> (24.1532, -56.5346) centre (24.1532, -54.5346) ccw
  line L12 (27.0881, -59.4916) -> (13.6537, -59.4916)
  arc A16 (24.1532, -52.5346) -> (24.1532, -56.5346) centre (24.1532, -54.5346) ccw
  line L13 (37.5876, -52.5346) -> (24.1532, -52.5346)
  arc A17 (37.5876, -56.5346) -> (37.5876, -52.5346) centre (37.5876, -54.5346) ccw
  line L14 (24.1532, -56.5346) -> (37.5876, -56.5346)
  line L15 (-6.3463, -63.4916) -> (7.0881, -63.4916)
  line L16 (7.0881, -59.4916) -> (-6.3463, -59.4916)
  arc A18 (4.1532, -52.5346) -> (4.1532, -56.5346) centre (4.1532, -54.5346) ccw
  arc A19 (7.0881, -63.4916) -> (7.0881, -59.4916) centre (7.0881, -61.4916) ccw
  arc A20 (13.6537, -59.4916) -> (13.6537, -63.4916) centre (13.6537, -61.4916) ccw
  line L17 (17.5876, -52.5346) -> (4.1532, -52.5346)
  line L18 (4.1532, -56.5346) -> (17.5876, -56.5346)
  arc A21 (17.5876, -56.5346) -> (17.5876, -52.5346) centre (17.5876, -54.5346) ccw
  line L19 (13.6537, -63.4916) -> (27.0881, -63.4916)
  arc A22 (-26.3463, -59.4916) -> (-26.3463, -63.4916) centre (-26.3463, -61.4916) ccw
  arc A23 (7.0881, -63.4916) -> (7.0881, -59.4916) centre (7.0881, -61.4916) ccw
  arc A24 (4.1532, -52.5346) -> (4.1532, -56.5346) centre (4.1532, -54.5346) ccw
  line L20 (7.0881, -59.4916) -> (-6.3463, -59.4916)
  arc A25 (4.1532, -52.5346) -> (4.1532, -56.5346) centre (4.1532, -54.5346) ccw
  line L21 (17.5876, -52.5346) -> (4.1532, -52.5346)
  arc A26 (17.5876, -56.5346) -> (17.5876, -52.5346) centre (17.5876, -54.5346) ccw
  line L22 (4.1532, -56.5346) -> (17.5876, -56.5346)
  line L23 (-26.3463, -63.4916) -> (-12.9119, -63.4916)
  line L24 (-12.9119, -59.4916) -> (-26.3463, -59.4916)
  arc A27 (-15.8468, -52.5346) -> (-15.8468, -56.5346) centre (-15.8468, -54.5346) ccw
  arc A28 (-12.9119, -63.4916) -> (-12.9119, -59.4916) centre (-12.9119, -61.4916) ccw
  arc A29 (-6.3463, -59.4916) -> (-6.3463, -63.4916) centre (-6.3463, -61.4916) ccw
  line L25 (-2.4124, -52.5346) -> (-15.8468, -52.5346)
  line L26 (-15.8468, -56.5346) -> (-2.4124, -56.5346)
  arc A30 (-2.4124, -56.5346) -> (-2.4124, -52.5346) centre (-2.4124, -54.5346) ccw
  line L27 (-6.3463, -63.4916) -> (7.0881, -63.4916)
  arc A31 (-46.3463, -59.4916) -> (-46.3463, -63.4916) centre (-46.3463, -61.4916) ccw
  arc A32 (-12.9119, -63.4916) -> (-12.9119, -59.4916) centre (-12.9119, -61.4916) ccw
  arc A33 (-15.8468, -52.5346) -> (-15.8468, -56.5346) centre (-15.8468, -54.5346) ccw
  line L28 (-12.9119, -59.4916) -> (-26.3463, -59.4916)
  arc A34 (-15.8468, -52.5346) -> (-15.8468, -56.5346) centre (-15.8468, -54.5346) ccw
  line L29 (-2.4124, -52.5346) -> (-15.8468, -52.5346)
  arc A35 (-2.4124, -56.5346) -> (-2.4124, -52.5346) centre (-2.4124, -54.5346) ccw
  line L30 (-15.8468, -56.5346) -> (-2.4124, -56.5346)
  line L31 (-46.3463, -63.4916) -> (-32.9119, -63.4916)
  line L32 (-32.9119, -59.4916) -> (-46.3463, -59.4916)
  arc A36 (-35.8468, -52.5346) -> (-35.8468, -56.5346) centre (-35.8468, -54.5346) ccw
  arc A37 (-32.9119, -63.4916) -> (-32.9119, -59.4916) centre (-32.9119, -61.4916) ccw
  arc A38 (-26.3463, -59.4916) -> (-26.3463, -63.4916) centre (-26.3463, -61.4916) ccw
  line L33 (-22.4124, -52.5346) -> (-35.8468, -52.5346)
  line L34 (-35.8468, -56.5346) -> (-22.4124, -56.5346)
  arc A39 (-22.4124, -56.5346) -> (-22.4124, -52.5346) centre (-22.4124, -54.5346) ccw
  line L35 (-26.3463, -63.4916) -> (-12.9119, -63.4916)
  arc A40 (-66.3463, -59.4916) -> (-66.3463, -63.4916) centre (-66.3463, -61.4916) ccw
  arc A41 (-32.9119, -63.4916) -> (-32.9119, -59.4916) centre (-32.9119, -61.4916) ccw
  arc A42 (-35.8468, -52.5346) -> (-35.8468, -56.5346) centre (-35.8468, -54.5346) ccw
  line L36 (-32.9119, -59.4916) -> (-46.3463, -59.4916)
  arc A43 (-35.8468, -52.5346) -> (-35.8468, -56.5346) centre (-35.8468, -54.5346) ccw
  line L37 (-22.4124, -52.5346) -> (-35.8468, -52.5346)
  arc A44 (-22.4124, -56.5346) -> (-22.4124, -52.5346) centre (-22.4124, -54.5346) ccw
  line L38 (-35.8468, -56.5346) -> (-22.4124, -56.5346)
  line L39 (-66.3463, -63.4916) -> (-52.9119, -63.4916)
  line L40 (-52.9119, -59.4916) -> (-66.3463, -59.4916)
  arc A45 (-55.8468, -52.5346) -> (-55.8468, -56.5346) centre (-55.8468, -54.5346) ccw
  arc A46 (-52.9119, -63.4916) -> (-52.9119, -59.4916) centre (-52.9119, -61.4916) ccw
  arc A47 (-46.3463, -59.4916) -> (-46.3463, -63.4916) centre (-46.3463, -61.4916) ccw
  line L41 (-42.4124, -52.5346) -> (-55.8468, -52.5346)
  line L42 (-55.8468, -56.5346) -> (-42.4124, -56.5346)
  arc A48 (-42.4124, -56.5346) -> (-42.4124, -52.5346) centre (-42.4124, -54.5346) ccw
  line L43 (-46.3463, -63.4916) -> (-32.9119, -63.4916)
  arc A49 (-86.3463, -59.4916) -> (-86.3463, -63.4916) centre (-86.3463, -61.4916) ccw
  arc A50 (-52.9119, -63.4916) -> (-52.9119, -59.4916) centre (-52.9119, -61.4916) ccw
  arc A51 (-55.8468, -52.5346) -> (-55.8468, -56.5346) centre (-55.8468, -54.5346) ccw
  line L44 (-52.9119, -59.4916) -> (-66.3463, -59.4916)
  arc A52 (-55.8468, -52.5346) -> (-55.8468, -56.5346) centre (-55.8468, -54.5346) ccw
  line L45 (-42.4124, -52.5346) -> (-55.8468, -52.5346)
  arc A53 (-42.4124, -56.5346) -> (-42.4124, -52.5346) centre (-42.4124, -54.5346) ccw
  line L46 (-55.8468, -56.5346) -> (-42.4124, -56.5346)
  line L47 (-86.3463, -63.4916) -> (-72.9119, -63.4916)
  line L48 (-72.9119, -59.4916) -> (-86.3463, -59.4916)
  arc A54 (-75.8468, -52.5346) -> (-75.8468, -56.5346) centre (-75.8468, -54.5346) ccw
  arc A55 (-72.9119, -63.4916) -> (-72.9119, -59.4916) centre (-72.9119, -61.4916) ccw
  arc A56 (-66.3463, -59.4916) -> (-66.3463, -63.4916) centre (-66.3463, -61.4916) ccw
  line L49 (-62.4124, -52.5346) -> (-75.8468, -52.5346)
  line L50 (-75.8468, -56.5346) -> (-62.4124, -56.5346)
  arc A57 (-62.4124, -56.5346) -> (-62.4124, -52.5346) centre (-62.4124, -54.5346) ccw
  line L51 (-66.3463, -63.4916) -> (-52.9119, -63.4916)
  arc A58 (-106.3463, -59.4916) -> (-106.3463, -63.4916) centre (-106.3463, -61.4916) ccw
  arc A59 (-72.9119, -63.4916) -> (-72.9119, -59.4916) centre (-72.9119, -61.4916) ccw
  arc A60 (-75.8468, -52.5346) -> (-75.8468, -56.5346) centre (-75.8468, -54.5346) ccw
  line L52 (-72.9119, -59.4916) -> (-86.3463, -59.4916)
  arc A61 (-75.8468, -52.5346) -> (-75.8468, -56.5346) centre (-75.8468, -54.5346) ccw
  line L53 (-62.4124, -52.5346) -> (-75.8468, -52.5346)
  arc A62 (-62.4124, -56.5346) -> (-62.4124, -52.5346) centre (-62.4124, -54.5346) ccw
  line L54 (-75.8468, -56.5346) -> (-62.4124, -56.5346)
  line L55 (-106.3463, -63.4916) -> (-92.9119, -63.4916)
  line L56 (-92.9119, -59.4916) -> (-106.3463, -59.4916)
  arc A63 (-95.8468, -52.5346) -> (-95.8468, -56.5346) centre (-95.8468, -54.5346) ccw
  arc A64 (-92.9119, -63.4916) -> (-92.9119, -59.4916) centre (-92.9119, -61.4916) ccw
  arc A65 (-86.3463, -59.4916) -> (-86.3463, -63.4916) centre (-86.3463, -61.4916) ccw
  line L57 (-82.4124, -52.5346) -> (-95.8468, -52.5346)
  line L58 (-95.8468, -56.5346) -> (-82.4124, -56.5346)
  arc A66 (-82.4124, -56.5346) -> (-82.4124, -52.5346) centre (-82.4124, -54.5346) ccw
  line L59 (-86.3463, -63.4916) -> (-72.9119, -63.4916)
  arc A67 (33.6537, -59.4916) -> (33.6537, -63.4916) centre (33.6537, -61.4916) ccw
  arc A68 (67.0881, -63.4916) -> (67.0881, -59.4916) centre (67.0881, -61.4916) ccw
  arc A69 (64.1532, -52.5346) -> (64.1532, -56.5346) centre (64.1532, -54.5346) ccw
  line L60 (67.0881, -59.4916) -> (53.6537, -59.4916)
  arc A70 (64.1532, -52.5346) -> (64.1532, -56.5346) centre (64.1532, -54.5346) ccw
  line L61 (77.5876, -52.5346) -> (64.1532, -52.5346)
  arc A71 (77.5876, -56.5346) -> (77.5876, -52.5346) centre (77.5876, -54.5346) ccw
  line L62 (64.1532, -56.5346) -> (77.5876, -56.5346)
  line L63 (33.6537, -63.4916) -> (47.0881, -63.4916)
  line L64 (47.0881, -59.4916) -> (33.6537, -59.4916)
  arc A72 (44.1532, -52.5346) -> (44.1532, -56.5346) centre (44.1532, -54.5346) ccw
  arc A73 (47.0881, -63.4916) -> (47.0881, -59.4916) centre (47.0881, -61.4916) ccw
  arc A74 (53.6537, -59.4916) -> (53.6537, -63.4916) centre (53.6537, -61.4916) ccw
  line L65 (57.5876, -52.5346) -> (44.1532, -52.5346)
  line L66 (44.1532, -56.5346) -> (57.5876, -56.5346)
  arc A75 (57.5876, -56.5346) -> (57.5876, -52.5346) centre (57.5876, -54.5346) ccw
  line L67 (53.6537, -63.4916) -> (67.0881, -63.4916)
  arc A76 (13.6537, -59.4916) -> (13.6537, -63.4916) centre (13.6537, -61.4916) ccw
  arc A77 (47.0881, -63.4916) -> (47.0881, -59.4916) centre (47.0881, -61.4916) ccw
  arc A78 (44.1532, -52.5346) -> (44.1532, -56.5346) centre (44.1532, -54.5346) ccw
  line L68 (47.0881, -59.4916) -> (33.6537, -59.4916)
  arc A79 (44.1532, -52.5346) -> (44.1532, -56.5346) centre (44.1532, -54.5346) ccw
  line L69 (57.5876, -52.5346) -> (44.1532, -52.5346)
  arc A80 (57.5876, -56.5346) -> (57.5876, -52.5346) centre (57.5876, -54.5346) ccw
  line L70 (44.1532, -56.5346) -> (57.5876, -56.5346)
  line L71 (13.6537, -63.4916) -> (27.0881, -63.4916)
  line L72 (27.0881, -59.4916) -> (13.6537, -59.4916)
  arc A81 (24.1532, -52.5346) -> (24.1532, -56.5346) centre (24.1532, -54.5346) ccw
  arc A82 (27.0881, -63.4916) -> (27.0881, -59.4916) centre (27.0881, -61.4916) ccw
  arc A83 (33.6537, -59.4916) -> (33.6537, -63.4916) centre (33.6537, -61.4916) ccw
  line L73 (37.5876, -52.5346) -> (24.1532, -52.5346)
  line L74 (24.1532, -56.5346) -> (37.5876, -56.5346)
  arc A84 (37.5876, -56.5346) -> (37.5876, -52.5346) centre (37.5876, -54.5346) ccw
  line L75 (33.6537, -63.4916) -> (47.0881, -63.4916)
  arc A85 (-6.3463, -59.4916) -> (-6.3463, -63.4916) centre (-6.3463, -61.4916) ccw
  arc A86 (27.0881, -63.4916) -> (27.0881, -59.4916) centre (27.0881, -61.4916) ccw
  arc A87 (24.1532, -52.5346) -> (24.1532, -56.5346) centre (24.1532, -54.5346) ccw
  line L76 (27.0881, -59.4916) -> (13.6537, -59.4916)
  arc A88 (24.1532, -52.5346) -> (24.1532, -56.5346) centre (24.1532, -54.5346) ccw
  line L77 (37.5876, -52.5346) -> (24.1532, -52.5346)
  arc A89 (37.5876, -56.5346) -> (37.5876, -52.5346) centre (37.5876, -54.5346) ccw
  line L78 (24.1532, -56.5346) -> (37.5876, -56.5346)
  line L79 (-6.3463, -63.4916) -> (7.0881, -63.4916)
  line L80 (7.0881, -59.4916) -> (-6.3463, -59.4916)
  arc A90 (4.1532, -52.5346) -> (4.1532, -56.5346) centre (4.1532, -54.5346) ccw
  arc A91 (7.0881, -63.4916) -> (7.0881, -59.4916) centre (7.0881, -61.4916) ccw
  arc A92 (13.6537, -59.4916) -> (13.6537, -63.4916) centre (13.6537, -61.4916) ccw
  line L81 (17.5876, -52.5346) -> (4.1532, -52.5346)
  line L82 (4.1532, -56.5346) -> (17.5876, -56.5346)
  arc A93 (17.5876, -56.5346) -> (17.5876, -52.5346) centre (17.5876, -54.5346) ccw
  line L83 (13.6537, -63.4916) -> (27.0881, -63.4916)
  arc A94 (-26.3463, -59.4916) -> (-26.3463, -63.4916) centre (-26.3463, -61.4916) ccw
  arc A95 (7.0881, -63.4916) -> (7.0881, -59.4916) centre (7.0881, -61.4916) ccw
  arc A96 (4.1532, -52.5346) -> (4.1532, -56.5346) centre (4.1532, -54.5346) ccw
  line L84 (7.0881, -59.4916) -> (-6.3463, -59.4916)
  arc A97 (4.1532, -52.5346) -> (4.1532, -56.5346) centre (4.1532, -54.5346) ccw
  line L85 (17.5876, -52.5346) -> (4.1532, -52.5346)
  arc A98 (17.5876, -56.5346) -> (17.5876, -52.5346) centre (17.5876, -54.5346) ccw
  line L86 (4.1532, -56.5346) -> (17.5876, -56.5346)
  line L87 (-26.3463, -63.4916) -> (-12.9119, -63.4916)
  line L88 (-12.9119, -59.4916) -> (-26.3463, -59.4916)
  arc A99 (-15.8468, -52.5346) -> (-15.8468, -56.5346) centre (-15.8468, -54.5346) ccw
  arc A100 (-12.9119, -63.4916) -> (-12.9119, -59.4916) centre (-12.9119, -61.4916) ccw
  arc A101 (-6.3463, -59.4916) -> (-6.3463, -63.4916) centre (-6.3463, -61.4916) ccw
  line L89 (-2.4124, -52.5346) -> (-15.8468, -52.5346)
  line L90 (-15.8468, -56.5346) -> (-2.4124, -56.5346)
  arc A102 (-2.4124, -56.5346) -> (-2.4124, -52.5346) centre (-2.4124, -54.5346) ccw
  line L91 (-6.3463, -63.4916) -> (7.0881, -63.4916)
  arc A103 (-46.3463, -59.4916) -> (-46.3463, -63.4916) centre (-46.3463, -61.4916) ccw
  arc A104 (-12.9119, -63.4916) -> (-12.9119, -59.4916) centre (-12.9119, -61.4916) ccw
  arc A105 (-15.8468, -52.5346) -> (-15.8468, -56.5346) centre (-15.8468, -54.5346) ccw
  line L92 (-12.9119, -59.4916) -> (-26.3463, -59.4916)
  arc A106 (-15.8468, -52.5346) -> (-15.8468, -56.5346) centre (-15.8468, -54.5346) ccw
  line L93 (-2.4124, -52.5346) -> (-15.8468, -52.5346)
  arc A107 (-2.4124, -56.5346) -> (-2.4124, -52.5346) centre (-2.4124, -54.5346) ccw
  line L94 (-15.8468, -56.5346) -> (-2.4124, -56.5346)
  line L95 (-46.3463, -63.4916) -> (-32.9119, -63.4916)
  line L96 (-32.9119, -59.4916) -> (-46.3463, -59.4916)
  arc A108 (-35.8468, -52.5346) -> (-35.8468, -56.5346) centre (-35.8468, -54.5346) ccw
  arc A109 (-32.9119, -63.4916) -> (-32.9119, -59.4916) centre (-32.9119, -61.4916) ccw
  arc A110 (-26.3463, -59.4916) -> (-26.3463, -63.4916) centre (-26.3463, -61.4916) ccw
  line L97 (-22.4124, -52.5346) -> (-35.8468, -52.5346)
  line L98 (-35.8468, -56.5346) -> (-22.4124, -56.5346)
  arc A111 (-22.4124, -56.5346) -> (-22.4124, -52.5346) centre (-22.4124, -54.5346) ccw
  line L99 (-26.3463, -63.4916) -> (-12.9119, -63.4916)
  arc A112 (-66.3463, -59.4916) -> (-66.3463, -63.4916) centre (-66.3463, -61.4916) ccw
  arc A113 (-32.9119, -63.4916) -> (-32.9119, -59.4916) centre (-32.9119, -61.4916) ccw
  arc A114 (-35.8468, -52.5346) -> (-35.8468, -56.5346) centre (-35.8468, -54.5346) ccw
  line L100 (-32.9119, -59.4916) -> (-46.3463, -59.4916)
  arc A115 (-35.8468, -52.5346) -> (-35.8468, -56.5346) centre (-35.8468, -54.5346) ccw
  line L101 (-22.4124, -52.5346) -> (-35.8468, -52.5346)
  arc A116 (-22.4124, -56.5346) -> (-22.4124, -52.5346) centre (-22.4124, -54.5346) ccw
  line L102 (-35.8468, -56.5346) -> (-22.4124, -56.5346)
  line L103 (-66.3463, -63.4916) -> (-52.9119, -63.4916)
  line L104 (-52.9119, -59.4916) -> (-66.3463, -59.4916)
  arc A117 (-55.8468, -52.5346) -> (-55.8468, -56.5346) centre (-55.8468, -54.5346) ccw
  arc A118 (-52.9119, -63.4916) -> (-52.9119, -59.4916) centre (-52.9119, -61.4916) ccw
  arc A119 (-46.3463, -59.4916) -> (-46.3463, -63.4916) centre (-46.3463, -61.4916) ccw
  line L105 (-42.4124, -52.5346) -> (-55.8468, -52.5346)
  line L106 (-55.8468, -56.5346) -> (-42.4124, -56.5346)
  arc A120 (-42.4124, -56.5346) -> (-42.4124, -52.5346) centre (-42.4124, -54.5346) ccw
  line L107 (-46.3463, -63.4916) -> (-32.9119, -63.4916)
  arc A121 (-86.3463, -59.4916) -> (-86.3463, -63.4916) centre (-86.3463, -61.4916) ccw
  arc A122 (-52.9119, -63.4916) -> (-52.9119, -59.4916) centre (-52.9119, -61.4916) ccw
  arc A123 (-55.8468, -52.5346) -> (-55.8468, -56.5346) centre (-55.8468, -54.5346) ccw
  line L108 (-52.9119, -59.4916) -> (-66.3463, -59.4916)
  arc A124 (-55.8468, -52.5346) -> (-55.8468, -56.5346) centre (-55.8468, -54.5346) ccw
  line L109 (-42.4124, -52.5346) -> (-55.8468, -52.5346)
  arc A125 (-42.4124, -56.5346) -> (-42.4124, -52.5346) centre (-42.4124, -54.5346) ccw
  line L110 (-55.8468, -56.5346) -> (-42.4124, -56.5346)
  line L111 (-86.3463, -63.4916) -> (-72.9119, -63.4916)
  line L112 (-72.9119, -59.4916) -> (-86.3463, -59.4916)
  arc A126 (-75.8468, -52.5346) -> (-75.8468, -56.5346) centre (-75.8468, -54.5346) ccw
  arc A127 (-72.9119, -63.4916) -> (-72.9119, -59.4916) centre (-72.9119, -61.4916) ccw
  arc A128 (-66.3463, -59.4916) -> (-66.3463, -63.4916) centre (-66.3463, -61.4916) ccw
  line L113 (-62.4124, -52.5346) -> (-75.8468, -52.5346)
  line L114 (-75.8468, -56.5346) -> (-62.4124, -56.5346)
  arc A129 (-62.4124, -56.5346) -> (-62.4124, -52.5346) centre (-62.4124, -54.5346) ccw
  line L115 (-66.3463, -63.4916) -> (-52.9119, -63.4916)
  arc A130 (53.6537, -59.4916) -> (53.6537, -63.4916) centre (53.6537, -61.4916) ccw
  arc A131 (87.0881, -63.4916) -> (87.0881, -59.4916) centre (87.0881, -61.4916) ccw
  arc A132 (84.1532, -52.5346) -> (84.1532, -56.5346) centre (84.1532, -54.5346) ccw
  line L116 (87.0881, -59.4916) -> (73.6537, -59.4916)
  arc A133 (84.1532, -52.5346) -> (84.1532, -56.5346) centre (84.1532, -54.5346) ccw
  line L117 (97.5876, -52.5346) -> (84.1532, -52.5346)
  arc A134 (97.5876, -56.5346) -> (97.5876, -52.5346) centre (97.5876, -54.5346) ccw
  line L118 (84.1532, -56.5346) -> (97.5876, -56.5346)
  line L119 (53.6537, -63.4916) -> (67.0881, -63.4916)
  line L120 (67.0881, -59.4916) -> (53.6537, -59.4916)
  arc A135 (64.1532, -52.5346) -> (64.1532, -56.5346) centre (64.1532, -54.5346) ccw
  arc A136 (67.0881, -63.4916) -> (67.0881, -59.4916) centre (67.0881, -61.4916) ccw
  arc A137 (73.6537, -59.4916) -> (73.6537, -63.4916) centre (73.6537, -61.4916) ccw
  line L121 (77.5876, -52.5346) -> (64.1532, -52.5346)
  line L122 (64.1532, -56.5346) -> (77.5876, -56.5346)
  arc A138 (77.5876, -56.5346) -> (77.5876, -52.5346) centre (77.5876, -54.5346) ccw
  line L123 (73.6537, -63.4916) -> (87.0881, -63.4916)
  arc A139 (33.6537, -59.4916) -> (33.6537, -63.4916) centre (33.6537, -61.4916) ccw
  arc A140 (67.0881, -63.4916) -> (67.0881, -59.4916) centre (67.0881, -61.4916) ccw
  arc A141 (64.1532, -52.5346) -> (64.1532, -56.5346) centre (64.1532, -54.5346) ccw
  line L124 (67.0881, -59.4916) -> (53.6537, -59.4916)
  arc A142 (64.1532, -52.5346) -> (64.1532, -56.5346) centre (64.1532, -54.5346) ccw
  line L125 (77.5876, -52.5346) -> (64.1532, -52.5346)
  arc A143 (77.5876, -56.5346) -> (77.5876, -52.5346) centre (77.5876, -54.5346) ccw
  line L126 (64.1532, -56.5346) -> (77.5876, -56.5346)
  line L127 (33.6537, -63.4916) -> (47.0881, -63.4916)
  line L128 (47.0881, -59.4916) -> (33.6537, -59.4916)
  arc A144 (44.1532, -52.5346) -> (44.1532, -56.5346) centre (44.1532, -54.5346) ccw
  arc A145 (47.0881, -63.4916) -> (47.0881, -59.4916) centre (47.0881, -61.4916) ccw
  arc A146 (53.6537, -59.4916) -> (53.6537, -63.4916) centre (53.6537, -61.4916) ccw
  line L129 (57.5876, -52.5346) -> (44.1532, -52.5346)
  line L130 (44.1532, -56.5346) -> (57.5876, -56.5346)
  arc A147 (57.5876, -56.5346) -> (57.5876, -52.5346) centre (57.5876, -54.5346) ccw
  line L131 (53.6537, -63.4916) -> (67.0881, -63.4916)
  arc A148 (13.6537, -59.4916) -> (13.6537, -63.4916) centre (13.6537, -61.4916) ccw
  arc A149 (47.0881, -63.4916) -> (47.0881, -59.4916) centre (47.0881, -61.4916) ccw
  arc A150 (44.1532, -52.5346) -> (44.1532, -56.5346) centre (44.1532, -54.5346) ccw